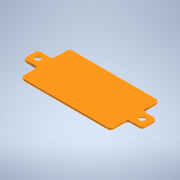
# Autodesk Inventor part: BatteryPlate
Saved by Autodesk Inventor 2021 (Build 250183000, 183)
## iProperties
Created: 2021-05-13
Part Number: BatteryPlate
Material: Generic
Document SubType Name: Modeling
Designer: ermoz
Density: 1 g/cm^3
Appearance: Default
Author: ermoz
Autodesk Inventor part; units mm, degrees
ref_plane "YZ Plane" through (0, 0, 0) normal (1, 0, 0) x (0, 1, 0)
ref_plane "XZ Plane" through (0, 0, 0) normal (0, 1, 0) x (-1, 0, 0)
ref_plane "XY Plane" through (0, 0, 0) normal (0, 0, 1) x (1, 0, 0)
sketch "Sketch1" plane through (0, 0, 0) normal (0, 1, 0) x (-1, 0, 0)
  line L0 (-31, -16.75) -> (31, -16.75)
  line L1 (31, -16.75) -> (31, 16.75)
  line L2 (31, 16.75) -> (-31, 16.75)
  line L3 (-31, 16.75) -> (-31, -16.75)
  line L4 (-31, -16.75) -> (31, 16.75) construction
  line L5 (31, -16.75) -> (-31, 16.75) construction
  point P0 (0, 0)
  dimension "d0" = 33.5
  dimension "d1" = 62
  constraints: 12 end point, 2 midpoint, 2 parallel, 1 horizontal, 1 perpendicular
  measures "d0" distance of L0.end L1.end
  measures "d1" distance of L1.end L2.end
extrude "Extrusion1" add sketch "Sketch1" along normal blind 1.5
fillet "Fillet1" radius 2 4 edges at (31, 0.75, 16.75) (31, 0.75, -16.75) (-31, 0.75, -16.75) (-31, 0.75, 16.75)
sketch "Sketch5" plane through (0, 0, 0) normal (0, -1, 0) x (1, 0, 0)
  line L0 (41, -5) -> (31, -5)
  line L1 (31, -5) -> (31, 5)
  line L2 (31, 5) -> (41, 5)
  line L3 (41, 5) -> (41, -5)
  line L4 (41, -5) -> (31, 5) construction
  line L5 (31, -5) -> (41, 5) construction
  line L6 (31, 14.75) -> (31, -14.75) projected
  line L7 (-41, -5) -> (-31, -5)
  line L8 (-31, -5) -> (-31, 5)
  line L9 (-31, 5) -> (-41, 5)
  line L10 (-41, 5) -> (-41, -5)
  line L11 (-41, -5) -> (-31, 5) construction
  line L12 (-31, -5) -> (-41, 5) construction
  line L13 (-31, -14.75) -> (-31, 14.75) projected
  point P0 (0, 0)
  point P1 (36, 0)
  point P2 (36, 0)
  point P3 (-36, 0)
  point P4 (-36, 0)
  dimension "d37" = 10
  dimension "d38" = 10
  constraints: 24 end point, 6 midpoint, 4 collinear, 4 parallel, 2 horizontal, 2 horizontal alignment, 2 perpendicular
  measures "d37" distance of L2.end L0.start
  measures "d38" distance of L0.start L0.end
extrude "Extrusion6" add sketch "Sketch5" against normal up to surface (1.5 mm away)
sketch "Sketch6" plane through (0, 0, 0) normal (0, -1, 0) x (1, 0, 0)
  circle A0 centre (36, 0) radius 1.75
  line L0 (31, 14.75) -> (31, 5) projected
  circle A1 centre (-36, 0) radius 1.75
  line L1 (-31, 5) -> (-31, 14.75) projected
  point P0 (0, 0)
  dimension "d41" = 3.5
  dimension "d42" = 5
  dimension "d51" = 5
  constraints: 2 centre point, 1 equal radius
  measures "d41" diameter of A0
  measures "d42" distance from line of L0 A0.centre
  measures "d51" distance from line of L1 A1.centre
extrude "Extrusion7" cut sketch "Sketch6" against normal up to surface (1.5 mm away)
fillet "Fillet6" radius 2 8 edges at (31, 0.75, 5) (41, 0.75, 5) (41, 0.75, -5) (31, 0.75, -5) (-31, 0.75, 5) (-41, 0.75, 5) (-41, 0.75, -5) (-31, 0.75, -5)
chamfer "Chamfer1" distance 1.5 angle 45 2 edges at (34.25, 0, 0) (-37.75, 0, 0)
equation "\"d51\" = d42"
body "Solid1"
